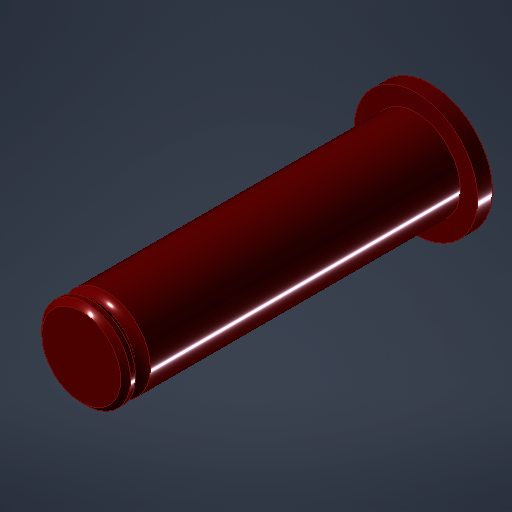
# Autodesk Inventor part: Long Pin
Saved by Autodesk Inventor 2026.2 (Build 302298010, 298A)
## iProperties
Created: 2026-05-31
Part Number: Long Pin
Material: Generic
Document SubType Name: Modeling
Designer: yassi
Density: 1 g/cm^3
Appearance: Light Red
Author: yassi
## iProperties of the stored document Long Pin_3DPrint.ipt
Created: 2026-06-01
Part Number: Long Pin_3DPrint
Material: Generic
Document SubType Name: Modeling
Designer: yassi
Density: 1 g/cm^3
Appearance: Default
Author: yassi
Autodesk Inventor part; units mm, degrees
ref_plane "YZ Plane" through (0, 0, 0) normal (1, 0, 0) x (0, 1, 0)
ref_plane "XZ Plane" through (0, 0, 0) normal (0, 1, 0) x (-1, 0, 0)
ref_plane "XY Plane" through (0, 0, 0) normal (0, 0, 1) x (1, 0, 0)
sketch "Sketch1" plane through (0, 0, 0) normal (0, 0, 1) x (1, 0, 0)
  circle A0 centre (0, 0) radius 6.25
  dimension "d0" = 12.5
  constraints: 1 centre point, 1 coincident
  measures "d0" diameter of A0
extrude "Extrusion1" add sketch "Sketch1" along normal blind 1.5
sketch "Sketch2" plane through (0, 0, 1.5) normal (0, 0, 1) x (1, 0, 0)
  circle A0 centre (0, 0) radius 6.25 projected
  circle A1 centre (0, 0) radius 4.5
  dimension "d3" = 9
  constraints: 1 centre point, 1 coincident
  measures "d3" diameter of A1
extrude "Extrusion2" add sketch "Sketch2" along normal blind 31.4 contours A1
sketch "Sketch3" plane through (0, 0, 32.9) normal (0, 0, 1) x (1, 0, 0)
  circle A0 centre (0, 0) radius 4.5 projected
  circle A1 centre (0, 0) radius 3.75
  dimension "d6" = 7.5
  constraints: 1 centre point, 1 coincident
  measures "d6" diameter of A1
extrude "Extrusion3" add sketch "Sketch3" along normal blind 0.75 contours A1
fillet "Fillet1" radius 2 1 edges at (-3.75, 0, 32.9)
sketch "Sketch4" plane through (0, 0, 33.65) normal (0, 0, 1) x (1, 0, 0)
  circle A0 centre (0, 0) radius 4.5
  dimension "d10" = 9
  constraints: 1 centre point, 1 coincident
  measures "d10" diameter of A0
extrude "Extrusion4" add sketch "Sketch4" along normal blind 0.75
fillet "Fillet2" radius 2 1 edges at (-4.5, 0, 33.65)
sketch "Sketch5" plane through (0, 0, 34.4) normal (0, 0, 1) x (1, 0, 0)
  circle A0 centre (0, 0) radius 4.5
  dimension "d14" = 9
  constraints: 1 centre point, 1 coincident
  measures "d14" diameter of A0
extrude "Extrusion5" add sketch "Sketch5" along normal blind 0.5
sketch "Sketch6" plane through (0, 0, 34.9) normal (0, 0, 1) x (1, 0, 0)
  circle A0 centre (0, 0) radius 4
  dimension "d17" = 8
  constraints: 1 centre point, 1 coincident
  measures "d17" diameter of A0
extrude "Extrusion6" add sketch "Sketch6" along normal blind 0.5
fillet "Fillet3" radius 3 1 edges at (-4, 0, 34.9)
body "Solid1"
